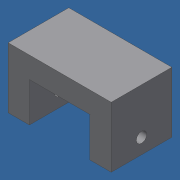
# Autodesk Inventor part: FanSpace
Saved by Autodesk Inventor 2021 (Build 250183000, 183)
## iProperties
Created: 2022-09-12
Part Number: FanSpace
Material: Generic
Document SubType Name: Modeling
Designer: Nathann
Density: 1 g/cm^3
Appearance: Default
Author: Nathann
Autodesk Inventor part; units mm, degrees
ref_plane "YZ Plane" through (0, 0, 0) normal (1, 0, 0) x (0, 1, 0)
ref_plane "XZ Plane" through (0, 0, 0) normal (0, 1, 0) x (-1, 0, 0)
ref_plane "XY Plane" through (0, 0, 0) normal (0, 0, 1) x (1, 0, 0)
sketch "Sketch1" plane through (0, 0, 0) normal (0, 0, 1) x (1, 0, 0)
  line L0 (0, 0) -> (7, 0)
  line L1 (7, 0) -> (7, 20)
  line L2 (7, 20) -> (0, 20)
  line L3 (0, 20) -> (0, 0)
  line L4 (7, 20) -> (27, 20)
  line L5 (27, 20) -> (27, 13)
  line L6 (27, 13) -> (7, 13)
  line L7 (7, 13) -> (7, 20)
  line L8 (27, 20) -> (34, 20)
  line L9 (34, 20) -> (34, 0)
  line L10 (34, 0) -> (27, 0)
  line L11 (27, 0) -> (27, 20)
  dimension "d0" = 34
  dimension "d1" = 7
  dimension "d2" = 7
  dimension "d3" = 7
  dimension "d4" = 13
  constraints: 24 end point, 6 parallel, 3 horizontal, 3 perpendicular, 1 point on line
  measures "d0" distance between parallel lines of L9 L3
  measures "d1" distance between parallel lines of L9 L11
  measures "d2" distance between parallel lines of L3 L1
  measures "d3" distance between parallel lines of L6 L4
  measures "d4" distance between parallel lines of L0 L6
extrude "Extrusion1" add sketch "Sketch1" along normal blind 20
sketch "Sketch2" plane through (7, 0, 0) normal (1, 0, 0) x (0, 0, -1)
  circle A0 centre (-10, 5) radius 2.5
  line L0 (-20, 0) -> (-20, 20) projected
  line L1 (0, 0) -> (-20, 0) projected
  dimension "d7" = 5
  dimension "d8" = 10
  dimension "d9" = 5
  constraints: 1 centre point
  measures "d7" diameter of A0
  measures "d8" distance from line of L0 A0.centre
  measures "d9" distance from line of L1 A0.centre
extrude "Extrusion2" cut sketch "Sketch2" along normal blind 60 and the other way blind 10
body "Solid1"
